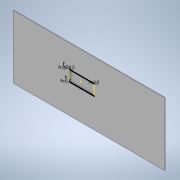
# Autodesk Inventor part: DecupajAgatare
Saved by Autodesk Inventor 2022 (Build 260153000, 153)
## iProperties
Created: 2022-04-13
Part Number: DecupajAgatare
Material: Generic
Document SubType Name: Sheet Metal
Designer: Janina
Density: 1 g/cm^3
Sheet Metal Rule: Default_mm
Appearance: Default
Author: Janina
Autodesk Inventor part; units mm, degrees
ref_plane "YZ Plane" through (0, 0, 0) normal (1, 0, 0) x (0, 1, 0)
ref_plane "XZ Plane" through (0, 0, 0) normal (0, 1, 0) x (-1, 0, 0)
ref_plane "XY Plane" through (0, 0, 0) normal (0, 0, 1) x (1, 0, 0)
sketch "Sketch1" plane through (0, 0, 0) normal (0, 0, 1) x (1, 0, 0)
  line L0 (-53.3333, 22.2222) -> (66.6667, 22.2222)
  line L1 (66.6667, 22.2222) -> (66.6667, -27.7778)
  line L2 (66.6667, -27.7778) -> (-53.3333, -27.7778)
  line L3 (-53.3333, -27.7778) -> (-53.3333, 22.2222)
  point P0 (0, 0)
  dimension "d0" = 120
  dimension "d1" = 50
  measures "d0" distance of L0.start L0.end
  measures "d1" distance of L0.end L1.end
extrude "Plate1" add sketch "Sketch1" along normal blind 0.5
sketch "Sketch2" plane through (0, 0, 0.5) normal (0, 0, 1) x (1, 0, 0)
  line L0 (-9.1667, 3.75) -> (10.8333, 3.75)
  line L1 (10.8333, 3.75) -> (10.8333, -4.25)
  line L2 (10.8333, -4.25) -> (-9.1667, -4.25)
  line L3 (-9.1667, -4.25) -> (-9.1667, 3.75)
  point P0 (0, 0)
  point P1 (0.8333, -0.25)
  dimension "d3" = 20
  dimension "d4" = 8
  dimension "d5" = 10
  dimension "d6" = 4
  constraints: 8 end point, 2 parallel, 1 horizontal, 1 perpendicular
  measures "d3" distance of L0.start L0.end
  measures "d4" distance of L0.end L1.end
  measures "d5" distance from line of L3 point (0.833, -0.25)
  measures "d6" distance from line of L2 point (0.833, -0.25)
extrude "Extrusion1" add sketch "Sketch2" against normal blind 1.5
sketch "Sketch3" plane through (0, 0, 0.5) normal (0, 0, 1) x (1, 0, 0)
  line L0 (-9.1667, -4.25) -> (-9.1667, 3.75) projected
  line L1 (10.8333, 3.75) -> (10.8333, -4.25) projected
  line L2 (-9.1667, -4.25) -> (10.8333, -4.25) projected
  line L3 (10.8333, 3.75) -> (-9.1667, 3.75) projected
  line L4 (10.3333, -4.25) -> (-8.6667, -4.25)
  line L5 (-8.6667, -4.25) -> (-8.6667, 3.75)
  line L6 (-8.6667, 3.75) -> (10.3333, 3.75)
  line L7 (10.3333, 3.75) -> (10.3333, -4.25)
  point P0 (0, 0)
  point P1 (-8.6667, -4.25)
  dimension "d11" = 0.5
  dimension "d12" = 0.5
  constraints: 8 end point, 2 collinear, 2 parallel, 1 horizontal, 1 perpendicular
  measures "d11" distance between parallel lines of L1 L7
  measures "d12" distance between parallel lines of L0 L5
extrude "Extrusion2" cut sketch "Sketch3" against normal blind 1 contours L5 L3 L7 L2
sketch "Sketch4" plane through (0, 0, 0.5) normal (0, 0, 1) x (1, 0, 0)
  line L0 (-8.6667, 3.75) -> (10.3333, 3.75) projected
  line L1 (-8.6667, -4.25) -> (-8.6667, 3.75) projected
  line L2 (10.3333, -4.25) -> (-8.6667, -4.25) projected
  line L3 (10.3333, 3.75) -> (10.3333, -4.25) projected
  line L4 (-9.1667, 4.25) -> (10.8333, 4.25)
  line L5 (10.8333, 4.25) -> (10.8333, 3.75)
  line L6 (10.8333, 3.75) -> (-9.1667, 3.75)
  line L7 (-9.1667, 3.75) -> (-9.1667, 4.25)
  line L8 (-9.1667, -4.25) -> (10.8333, -4.25)
  line L9 (10.8333, -4.25) -> (10.8333, -4.75)
  line L10 (10.8333, -4.75) -> (-9.1667, -4.75)
  line L11 (-9.1667, -4.75) -> (-9.1667, -4.25)
  point P0 (0, 0)
  dimension "d15" = 0.5
  dimension "d16" = 0.5
  dimension "d17" = 0.5
  dimension "d18" = 0.5
  constraints: 16 end point, 4 parallel, 2 collinear, 2 horizontal, 2 perpendicular, 2 point on line
  measures "d15" distance between parallel lines of L1 L7
  measures "d16" distance between parallel lines of L3 L5
  measures "d17" distance of L6.end L4.start
  measures "d18" distance of L10.end L8.start
equation "\"d7\" = 3 * Thickness"
equation "\"d11\" = Thickness"
equation "\"d12\" = Thickness"
equation "\"d13\" = 2 * Thickness"
equation "\"d15\" = Thickness"
equation "\"d16\" = Thickness"
equation "\"d17\" = Thickness"
equation "\"d18\" = Thickness"
equation "\"d2\" = Thickness"
equation "\"BendRadius\" = Thickness"
equation "\"BendReliefWidth\" = Thickness"
equation "\"BendReliefDepth\" = 0.5 * Thickness"
equation "\"CornerReliefSize\" = 4 * Thickness"
equation "\"MinimumRemnant\" = 2 * Thickness"
equation "\"TransitionRadius\" = BendRadius"
equation "\"JacobiRadiusSize\" = BendRadius"
equation "\"GapSize\" = Thickness"
equation "\"Thickness\" = 0.5"
body "Solid1"
